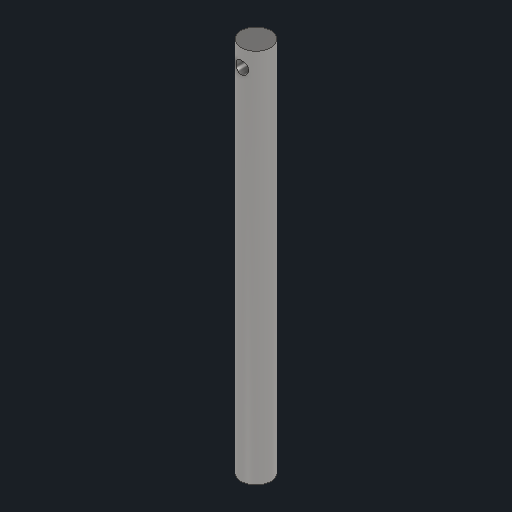
# Autodesk Inventor part: WashPistonRod
Saved by Autodesk Inventor 2024 (Build 280153000, 153)
## iProperties
Created: 2025-02-08
Part Number: WashPistonRod
Material: Stainless Steel
Document SubType Name: Modeling
Designer: Tommy Rohmann
Density: 8 g/cm^3
Appearance: Semi-Polished
Author: Tommy Rohmann
Autodesk Inventor part; units mm, degrees
ref_plane "YZ Plane" through (0, 0, 0) normal (1, 0, 0) x (0, 1, 0)
ref_plane "XZ Plane" through (0, 0, 0) normal (0, 1, 0) x (-1, 0, 0)
ref_plane "XY Plane" through (0, 0, 0) normal (0, 0, 1) x (1, 0, 0)
sketch "WashPistonRod" plane through (0, 0, 0) normal (0, 0, 1) x (1, 0, 0)
  line L0 (107.6058, 55.204) -> (118.7183, 55.204)
  line L1 (118.7183, 55.204) -> (118.7183, 334.858)
  line L2 (107.6058, 55.204) -> (107.6058, 334.858)
  line L3 (118.7183, 334.858) -> (107.6058, 334.858)
  circle A0 centre (107.6058, 322.158) radius 4.7625
  point P0 (113.1621, 176.283)
  dimension "d139" = 22.225
  dimension "d155" = 9.525
  dimension "d156" = 12.7
  dimension "d432" = 279.654
  measures "d139" diameter of L1 L2
  measures "d155" diameter of A0
  measures "d156" distance from line of L3 A0.centre
  measures "d432" distance of L0.end L1.end
derived "LAYOUT.ipt"
sketch "Sketch1" plane through (0, 0, 0) normal (0, 0, 1) x (1, 0, 0)
  line L0 (107.6058, 55.204) -> (118.7183, 55.204)
  line L1 (118.7183, 55.204) -> (118.7183, 334.858)
  line L2 (107.6058, 55.204) -> (107.6058, 334.858)
  line L3 (118.7183, 334.858) -> (107.6058, 334.858)
  circle A0 centre (107.6058, 322.158) radius 4.7625
revolve "Revolution1" add sketch "Sketch1" angle 360 about axis through (107.6058, 55.204, 0) along (0, 1, 0) picked at (109.8423, 322.354) contours L2 A0 L3 L1 L0 | L2 A0
extrude "Extrusion1" cut sketch "Sketch1" along normal mid plane 50.8 contours A0 L2 | L2 A0
body "Solid1"
